Autodesk Inventor part; units mm, degrees
(part 2 of 2)
  dimension "d200" = 50
  dimension "d201" = 40
  dimension "d202" = 20
  dimension "d203" = 50
  dimension "d204" = 40
  dimension "d205" = 20
  dimension "d206" = 50
  dimension "d207" = 20
  dimension "d208" = 40
  dimension "d209" = 50
  dimension "d210" = 40
  dimension "d211" = 20
  dimension "d212" = 50
  dimension "d213" = 40
  dimension "d214" = 20
  dimension "d215" = 50
  dimension "d216" = 40
  dimension "d217" = 20
  dimension "d218" = 50
  dimension "d219" = 40
  dimension "d220" = 20
  dimension "d221" = 50
  dimension "d222" = 20
  constraints: 534 end point, 121 parallel, 84 midpoint, 49 point on line, 43 perpendicular, 7 horizontal, 2 vertical
  measures "d159" distance of L49.end L48.end
  measures "d160" distance of L48.end L47.end
  measures "d161" distance from line of L41.start L50
  measures "d162" distance of L54.end L55.end
  measures "d163" distance of L53.end L54.end
  measures "d164" distance from line of L38.start L55
  measures "d165" distance of L60.end L61.end
  measures "d166" distance of L59.end L60.end
  measures "d167" distance from line of L37.end L59
  measures "d168" distance of L67.end L66.end
  measures "d169" distance of L66.end L65.end
  measures "d170" distance from line of L36.start L65
  measures "d171" distance of L73.end L72.end
  measures "d172" distance of L72.end L71.end
  measures "d173" distance from line of L35.start L73
  measures "d174" distance of L78.end L79.end
  measures "d175" distance of L77.end L78.end
  measures "d176" distance from line of L33.start L78
  measures "d177" distance of L86.end L85.end
  measures "d178" distance of L85.end L84.end
  measures "d179" distance from line of L32.start L84
  measures "d180" distance of L91.end L92.end
  measures "d181" distance of L90.end L91.end
  measures "d182" distance from line of L31.start L92
  measures "d183" distance of L97.end L98.end
  measures "d184" distance of L96.end L97.end
  measures "d185" distance from line of L29.start L99
  measures "d186" distance of L103.end L104.end
  measures "d187" distance of L102.end L103.end
  measures "d188" distance from line of L26.start L104
  measures "d189" distance of L109.end L110.end
  measures "d190" distance of L108.end L109.end
  measures "d191" distance from line of L25.start L111
  measures "d192" distance of L117.end L116.end
  measures "d193" distance of L116.end L115.end
  measures "d194" distance from line of L24.start L116
  measures "d195" distance of L123.end L122.end
  measures "d196" distance of L122.end L121.end
  measures "d197" distance from line of L21.start L122
  measures "d198" distance of L128.end L129.end
  measures "d199" distance of L127.end L128.end
  measures "d200" distance from line of L128 L22.start
  measures "d201" distance of L135.end L134.end
  measures "d202" distance of L134.end L133.end
  measures "d203" distance from line of L23.start L136
  measures "d204" distance of L140.end L141.end
  measures "d205" distance of L139.end L140.end
  measures "d206" distance from line of L20.start L142
  measures "d207" distance of L147.end L146.end
  measures "d208" distance of L146.end L145.end
  measures "d209" distance from line of L19.start L145
  measures "d210" distance of L155.end L154.end
  measures "d211" distance of L154.end L153.end
  measures "d212" distance from line of L42.start L156
  measures "d213" distance of L161.end L160.end
  measures "d214" distance of L160.end L159.end
  measures "d215" distance from line of L43.start L162
  measures "d216" distance of L167.end L168.end
  measures "d217" distance of L166.end L167.end
  measures "d218" distance from line of L44.start L167
  measures "d219" distance of L173.end L174.end
  measures "d220" distance of L172.end L173.end
  measures "d221" distance from line of L45.start L173
  measures "d222" distance of L179.end L180.end
extrude "Extrusão1" add sketch "Esboço5" along normal blind 0.2 contours L1 A3 L2 A4 L0 A14 L9 L11 A15 A16 A18 A17 L10 A1 A2 L8 A11 A12 A13 L3 A7 L7 A9 L5 A8 L6 A10 L4 A6 A5 A0 | A0 A5 A6 L4 A10 L6 A8 L5 A9 L7 A7 L3 A13 A12 A11 L8 A2 A1 L10 A17 A18 A16 A15 L11 L47 L35 A54 A55 A56 A38 L24 A39 A40 L25 A41 A42 A43 L26 A44 L27 A45 L28 A46 L29 A47 L30 A48 A49 A50 L31 A51 L32 A52 L33 A53 L34 L52 L9 A14 L0 A4 L2 A3 L1 | L52 L34 L56 L9 | L56 L34 L35 L47 | L58 L44 L56 L34 | L47 A68 L45 A67 A66 L46 L43 L51 A71 A70 L50 A69 L49 L35 | L35 L53 A72 L54 A73 A74 L55 L43 L46 A66 A67 L45 A68 L47 | L56 L44 L57 L34 | L58 L38 L56 L44 | L44 A63 L42 A64 A65 L43 L51 L36 A57 A58 L37 A59 L38 L58 | L56 L46 L43 L44 | L38 A59 L37 A58 A57 L36 | L36 L51 L43 L46
extrude "Extrusão2" add sketch "Esboço6" along normal blind 0.2
extrude "Extrusão3" add sketch "Esboço3" against normal blind 15 contours L3 L2 L1 L0 | L4 L5 L6 L7
